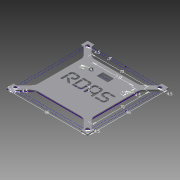
# Autodesk Inventor part: BattHolder
Saved by Autodesk Inventor 2014 SP1 (Build 180222100, 222)
## iProperties
Created: 2015-03-30
Part Number: BattHolder
Material: Generic
Document SubType Name: Modeling
Designer: Erin
Density: 1 g/cm^3
Appearance: Default
Author: Erin
Autodesk Inventor part; units mm, degrees
ref_plane "YZ Plane" through (0, 0, 0) normal (1, 0, 0) x (0, 1, 0)
ref_plane "XZ Plane" through (0, 0, 0) normal (0, 1, 0) x (-1, 0, 0)
ref_plane "XY Plane" through (0, 0, 0) normal (0, 0, 1) x (1, 0, 0)
sketch "Sketch1" plane through (0, 0, 0) normal (0, 0, 1) x (1, 0, 0)
  line L0 (-48, 48) -> (48, 48) construction
  line L1 (48, 48) -> (48, -48) construction
  line L2 (48, -48) -> (-48, -48) construction
  line L3 (-48, -48) -> (-48, 48) construction
  circle A0 centre (-45, 45) radius 2.25
  circle A1 centre (45, 45) radius 2.25
  line L4 (45, 45) -> (-45, 45) construction
  line L5 (-45, 45) -> (-45, -45) construction
  line L6 (-45, -45) -> (45, -45) construction
  line L7 (45, -45) -> (45, 45) construction
  circle A2 centre (45, -45) radius 2.25
  circle A3 centre (-45, -45) radius 2.25
  line L8 (-50.5, -50.5) -> (-42, -50.5)
  line L9 (-42, -50.5) -> (-42, -42)
  line L10 (-42, -42) -> (-50.5, -42)
  line L11 (-50.5, -42) -> (-50.5, -50.5)
  line L12 (0, 0) -> (-48, -48) construction
  line L13 (-35, 35) -> (35, 35)
  line L14 (35, 35) -> (35, -35)
  line L15 (35, -35) -> (-35, -35)
  line L16 (-35, -35) -> (-35, 35)
  line L17 (-2.4749, 2.4749) -> (2.4749, -2.4749)
  line L18 (2.4749, -2.4749) -> (-42.5251, -47.4749)
  line L19 (-42.5251, -47.4749) -> (-47.4749, -42.5251)
  line L20 (-47.4749, -42.5251) -> (-2.4749, 2.4749)
  line L21 (0, 0) -> (-45, -45) construction
  line L22 (-25, 30) -> (25, 30)
  line L23 (25, 30) -> (25, 15)
  line L24 (25, 15) -> (-25, 15)
  line L25 (-25, 15) -> (-25, 30)
  line L26 (-25, 22.5) -> (25, 22.5) construction
  circle A4 centre (-28, 22.1227) radius 2.25
  circle A5 centre (28, 22.1227) radius 2.25
  point P0 (0, 48)
  point P1 (48, 0)
  point P2 (35, 0)
  point P3 (0, 35)
  point P4 (0, 30)
  dimension "d0" = 96
  dimension "d1" = 96
  dimension "d2" = 4.5
  dimension "d3" = 4.5
  dimension "d4" = 3
  dimension "d5" = 4.5
  dimension "d6" = 4.5
  dimension "d9" = 3
  dimension "d10" = 3
  dimension "d11" = 70
  dimension "d12" = 70
  dimension "d13" = 7
  dimension "d14" = 0
  dimension "d23" = 5.5
  dimension "d24" = 5.5
  dimension "d27" = 15
  dimension "d28" = 50
  dimension "d29" = 4.5
  dimension "d30" = 4.5
  dimension "d31" = 3
  dimension "d32" = 3
  dimension "d33" = 5
  constraints: 54 end point, 12 parallel, 9 midpoint, 6 centre point, 6 perpendicular, 4 coincident, 4 horizontal, 3 vertical alignment, 2 horizontal alignment, 1 collinear, 3 other
  measures "d0" distance of L1.end L2.end
  measures "d1" distance of L0.end L1.end
  measures "d2" diameter of A0
  measures "d3" diameter of A1
  measures "d4" distance between parallel lines of L4 L0
  measures "d5" diameter of A2
  measures "d6" diameter of A3
  measures "d9" distance from line of A3.centre L10
  measures "d10" distance from line of A3.centre L9
  measures "d11" distance of L13.start L13.end
  measures "d12" distance of L13.end L14.end
  measures "d13" distance of L17.start L17.end
  measures "d14" distance from line of L5.end L19
  measures "d23" distance from line of L11 A3.centre
  measures "d24" distance from line of A3.centre L8
  measures "d27" distance of L22.end L23.end
  measures "d28" distance of L22.start L22.end
  measures "d29" diameter of A4
  measures "d30" diameter of A5
  measures "d31" distance from line of A4.centre L25
  measures "d32" distance from line of A5.centre L23
  measures "d33" distance between parallel lines of L22 L13
extrude "Extrusion1" add sketch "Sketch1" along normal blind 1.5 contours L20 L17 L18 L15 L16 | L16 L13 L14 L15 L18 L17 L20 | L22 L23 L24 L25 | A4 | A5
extrude "Extrusion2" add sketch "Sketch1" along normal blind 1.5 contours A3 L19 | A3 L19 L20 L10 L9 L18 | A3 L19 L18 L9 L8 L11 L10 L20 | L20 L16 L15 L18 L9 L10 | L20 L17 L18 L15 L16 picked at (-45.2318, -44.2867)
extrude "Extrusion3" cut sketch "Sketch1" along normal blind 10 contours A3 L19 | L19 A3
mirror "Mirror1" about plane through (0, 0, 0) normal (1, 0, 0) of "Extrusion2", "Extrusion3"
mirror "Mirror2" about plane through (0, 0, 0) normal (0, 1, 0) of "Extrusion2", "Extrusion3", "Mirror1"
fillet "Fillet2" radius 10 8 edges at (-35, -30.0503, 0.75) (-35, 30.0503, 0.75) (35, 30.0503, 0.75) (35, -30.0503, 0.75) (-30.0503, -35, 0.75) (30.0503, -35, 0.75) (30.0503, 35, 0.75) (-30.0503, 35, 0.75)
sketch "Sketch2" plane through (0, 0, 1.5) normal (0, 0, 1) x (1, 0, 0)
  line L0 (-28.3958, 7.9828) -> (28.458, 7.9828) construction
  line L1 (28.458, 7.9828) -> (28.458, -7.0172) construction
  line L2 (28.458, -7.0172) -> (-28.3958, -7.0172) construction
  line L3 (-28.3958, -7.0172) -> (-28.3958, 7.9828) construction
  line L4 (25.9081, 35) -> (-25.9081, 35) projected
  line L5 (-6.9, 26) -> (6.9, 26)
  line L6 (6.9, 26) -> (6.9, 18.2)
  line L7 (6.9, 18.2) -> (-6.9, 18.2)
  line L8 (-6.9, 18.2) -> (-6.9, 26)
  circle A0 centre (-16.9, 22.1) radius 2.9
  line L9 (-6.9, 22.1) -> (6.9, 22.1) construction
  spline S0 degree 2 poles (-17.7357, 2.8471) (-17.7357, 2.3566) (-18.4112, 1.6626) (-18.9202, 1.6626) knots 0 0 0 1 2 2 2
  line L10 (-18.9202, 1.6626) -> (-20.8912, 1.6626)
  line L11 (-20.8912, 1.6626) -> (-20.8912, -0.7063)
  line L12 (-20.8912, -0.7063) -> (-18.9202, -0.7063)
  spline S1 degree 2 poles (-18.9202, -0.7063) (-18.1892, -0.7063) (-16.8844, -0.1511) (-15.922, 0.8113) (-15.3668, 2.116) (-15.3668, 2.8471) knots 0 0 0 1 2 3 4 4 4
  line L13 (-15.3668, 2.8471) -> (-15.3668, 4.4294)
  spline S2 degree 2 poles (-15.3668, 4.4294) (-15.3668, 5.1605) (-15.922, 6.4652) (-16.8844, 7.4276) (-18.1892, 7.9828) (-18.9202, 7.9828) knots 0 0 0 1 2 3 4 4 4
  line L14 (-18.9202, 7.9828) -> (-20.8912, 7.9828)
  line L15 (-20.8912, 7.9828) -> (-20.8912, 5.6139)
  line L16 (-20.8912, 5.6139) -> (-18.9202, 5.6139)
  spline S3 degree 2 poles (-18.9202, 5.6139) (-18.4112, 5.6139) (-17.7357, 4.9199) (-17.7357, 4.4294) knots 0 0 0 1 2 2 2
  line L17 (-17.7357, 4.4294) -> (-17.7357, 2.8471)
  line L18 (-24.8425, -7.0172) -> (-27.2114, -7.0172)
  line L19 (-27.2114, -7.0172) -> (-27.2114, 1.6626)
  line L20 (-27.2114, 1.6626) -> (-24.8425, 1.6626)
  line L21 (-24.8425, 1.6626) -> (-24.8425, -7.0172)
  line L22 (-15.3668, -7.0172) -> (-15.3668, -6.5268)
  line L23 (-15.3668, -6.5268) -> (-21.03, -1.4928)
  line L24 (-21.03, -1.4928) -> (-24.0559, -1.4928)
  line L25 (-24.0559, -1.4928) -> (-24.0559, -1.9833)
  line L26 (-24.0559, -1.9833) -> (-18.365, -7.0172)
  line L27 (-18.365, -7.0172) -> (-15.3668, -7.0172)
  spline S4 degree 2 poles (-23.658, 5.6139) (-24.1484, 5.6139) (-24.8425, 4.9199) (-24.8425, 4.4294) knots 0 0 0 1 2 2 2
  line L28 (-24.8425, 4.4294) -> (-24.8425, 2.4584)
  line L29 (-24.8425, 2.4584) -> (-27.2114, 2.4584)
  line L30 (-27.2114, 2.4584) -> (-27.2114, 4.4294)
  spline S5 degree 2 poles (-27.2114, 4.4294) (-27.2114, 5.1605) (-26.6562, 6.4652) (-25.6938, 7.4276) (-24.389, 7.9828) (-23.658, 7.9828) knots 0 0 0 1 2 3 4 4 4
  line L31 (-23.658, 7.9828) -> (-21.687, 7.9828)
  line L32 (-21.687, 7.9828) -> (-21.687, 5.6139)
  line L33 (-21.687, 5.6139) -> (-23.658, 5.6139)
  spline S6 degree 2 poles (-4.7067, -4.6483) (-4.1978, -4.6483) (-3.5223, -3.9543) (-3.5223, -3.4639) knots 0 0 0 1 2 2 2
  line L34 (-3.5223, -3.4639) -> (-3.5223, 1.6719)
  line L35 (-3.5223, 1.6719) -> (-1.1534, 1.6719)
  line L36 (-1.1534, 1.6719) -> (-1.1534, -3.4639)
  spline S7 degree 2 poles (-1.1534, -3.4639) (-1.1534, -4.1949) (-1.7086, -5.4996) (-2.671, -6.462) (-3.9757, -7.0172) (-4.7067, -7.0172) knots 0 0 0 1 2 3 4 4 4
  line L37 (-4.7067, -7.0172) -> (-6.6777, -7.0172)
  line L38 (-6.6777, -7.0172) -> (-6.6777, -4.6483)
  line L39 (-6.6777, -4.6483) -> (-4.7067, -4.6483)
  line L40 (-12.9979, 4.8273) -> (-10.629, 4.8273)
  line L41 (-10.629, 4.8273) -> (-10.629, -3.8618)
  line L42 (-10.629, -3.8618) -> (-12.9979, -3.8618)
  line L43 (-12.9979, -3.8618) -> (-12.9979, 4.8273)
  spline S8 degree 2 poles (-3.5223, 4.4294) (-3.5223, 4.9199) (-4.1978, 5.6139) (-4.7067, 5.6139) knots 0 0 0 1 2 2 2
  line L44 (-4.7067, 5.6139) -> (-6.6777, 5.6139)
  line L45 (-6.6777, 5.6139) -> (-6.6777, 7.9828)
  line L46 (-6.6777, 7.9828) -> (-4.7067, 7.9828)
  spline S9 degree 2 poles (-4.7067, 7.9828) (-3.9757, 7.9828) (-2.671, 7.4276) (-1.7086, 6.4652) (-1.1534, 5.1605) (-1.1534, 4.4294) knots 0 0 0 1 2 3 4 4 4
  line L47 (-1.1534, 4.4294) -> (-1.1534, 2.4584)
  line L48 (-1.1534, 2.4584) -> (-3.5223, 2.4584)
  line L49 (-3.5223, 2.4584) -> (-3.5223, 4.4294)
  line L50 (-7.4735, 7.9828) -> (-7.4735, 5.6139)
  line L51 (-7.4735, 5.6139) -> (-12.9979, 5.6139)
  line L52 (-12.9979, 5.6139) -> (-12.9979, 7.9828)
  line L53 (-12.9979, 7.9828) -> (-7.4735, 7.9828)
  line L54 (-7.4735, -4.6483) -> (-7.4735, -7.0172)
  line L55 (-7.4735, -7.0172) -> (-12.9979, -7.0172)
  line L56 (-12.9979, -7.0172) -> (-12.9979, -4.6483)
  line L57 (-12.9979, -4.6483) -> (-7.4735, -4.6483)
  line L58 (6.7399, -1.4928) -> (6.7399, -3.8618)
  line L59 (6.7399, -3.8618) -> (4.7689, -3.8618)
  spline S10 degree 2 poles (4.7689, -3.8618) (4.2785, -3.8618) (3.5844, -4.5558) (3.5844, -5.0462) knots 0 0 0 1 2 2 2
  line L60 (3.5844, -5.0462) -> (3.5844, -7.0172)
  line L61 (3.5844, -7.0172) -> (1.2155, -7.0172)
  line L62 (1.2155, -7.0172) -> (1.2155, 1.6626)
  line L63 (1.2155, 1.6626) -> (3.5844, 1.6626)
  line L64 (3.5844, 1.6626) -> (3.5844, -0.3084)
  spline S11 degree 2 poles (3.5844, -0.3084) (3.5844, -0.7988) (4.2785, -1.4928) (4.7689, -1.4928) knots 0 0 0 1 2 2 2
  line L65 (4.7689, -1.4928) -> (6.7399, -1.4928)
  line L66 (7.5357, -3.8618) -> (7.5357, -1.4928)
  line L67 (7.5357, -1.4928) -> (9.5067, -1.4928)
  spline S12 degree 2 poles (9.5067, -1.4928) (10.0157, -1.4928) (10.6912, -0.7988) (10.6912, -0.3084) knots 0 0 0 1 2 2 2
  line L68 (10.6912, -0.3084) -> (10.6912, 1.6626)
  line L69 (10.6912, 1.6626) -> (13.0601, 1.6626)
  line L70 (13.0601, 1.6626) -> (13.0601, -7.0172)
  line L71 (13.0601, -7.0172) -> (10.6912, -7.0172)
  line L72 (10.6912, -7.0172) -> (10.6912, -5.0462)
  spline S13 degree 2 poles (10.6912, -5.0462) (10.6912, -4.5558) (10.0157, -3.8618) (9.5067, -3.8618) knots 0 0 0 1 2 2 2
  line L73 (9.5067, -3.8618) -> (7.5357, -3.8618)
  line L74 (3.5844, 2.4584) -> (1.2155, 2.4584)
  line L75 (1.2155, 2.4584) -> (1.2155, 4.4294)
  spline S14 degree 2 poles (1.2155, 4.4294) (1.2155, 5.1605) (1.7707, 6.4652) (2.7331, 7.4276) (4.0379, 7.9828) (4.7689, 7.9828) knots 0 0 0 1 2 3 4 4 4
  line L76 (4.7689, 7.9828) -> (6.7399, 7.9828)
  line L77 (6.7399, 7.9828) -> (6.7399, 5.6139)
  line L78 (6.7399, 5.6139) -> (4.7689, 5.6139)
  spline S15 degree 2 poles (4.7689, 5.6139) (4.2785, 5.6139) (3.5844, 4.9199) (3.5844, 4.4294) knots 0 0 0 1 2 2 2
  line L79 (3.5844, 4.4294) -> (3.5844, 2.4584)
  line L80 (7.5357, 5.6139) -> (7.5357, 7.9828)
  line L81 (7.5357, 7.9828) -> (9.5067, 7.9828)
  spline S16 degree 2 poles (9.5067, 7.9828) (10.2377, 7.9828) (11.5425, 7.4276) (12.5049, 6.4652) (13.0601, 5.1605) (13.0601, 4.4294) knots 0 0 0 1 2 3 4 4 4
  line L82 (13.0601, 4.4294) -> (13.0601, 2.4584)
  line L83 (13.0601, 2.4584) -> (10.6912, 2.4584)
  line L84 (10.6912, 2.4584) -> (10.6912, 4.4294)
  spline S17 degree 2 poles (10.6912, 4.4294) (10.6912, 4.9199) (10.0157, 5.6139) (9.5067, 5.6139) knots 0 0 0 1 2 2 2
  line L85 (9.5067, 5.6139) -> (7.5357, 5.6139)
  spline S18 degree 2 poles (24.9046, -3.4639) (24.9046, -3.9543) (24.2291, -4.6483) (23.7202, -4.6483) knots 0 0 0 1 2 2 2
  line L86 (23.7202, -4.6483) -> (21.7492, -4.6483)
  line L87 (21.7492, -4.6483) -> (21.7492, -7.0172)
  line L88 (21.7492, -7.0172) -> (23.7202, -7.0172)
  spline S19 degree 2 poles (23.7202, -7.0172) (24.4512, -7.0172) (25.7559, -6.462) (26.7183, -5.4996) (27.2735, -4.1949) (27.2735, -3.4639) knots 0 0 0 1 2 3 4 4 4
  line L89 (27.2735, -3.4639) -> (27.2735, -1.8815)
  spline S20 degree 2 poles (27.2735, -1.8815) (27.2735, -1.1505) (26.7183, 0.1543) (25.7559, 1.1167) (24.4512, 1.6719) (23.7202, 1.6719) knots 0 0 0 1 2 3 4 4 4
  line L90 (23.7202, 1.6719) -> (21.7492, 1.6719)
  line L91 (21.7492, 1.6719) -> (21.7492, -0.697)
  line L92 (21.7492, -0.697) -> (23.7202, -0.697)
  spline S21 degree 2 poles (23.7202, -0.697) (24.2291, -0.697) (24.9046, -1.3911) (24.9046, -1.8815) knots 0 0 0 1 2 2 2
  line L93 (24.9046, -1.8815) -> (24.9046, -3.4639)
  spline S22 degree 2 poles (17.7979, 4.4294) (17.7979, 4.9199) (18.4919, 5.6139) (18.9823, 5.6139) knots 0 0 0 1 2 2 2
  line L94 (18.9823, 5.6139) -> (20.9533, 5.6139)
  line L95 (20.9533, 5.6139) -> (20.9533, 7.9828)
  line L96 (20.9533, 7.9828) -> (18.9823, 7.9828)
  spline S23 degree 2 poles (18.9823, 7.9828) (18.2513, 7.9828) (16.9466, 7.4276) (15.9842, 6.4652) (15.429, 5.1605) (15.429, 4.4294) knots 0 0 0 1 2 3 4 4 4
  line L97 (15.429, 4.4294) -> (15.429, 2.8563)
  spline S24 degree 2 poles (15.429, 2.8563) (15.429, 2.1253) (15.9842, 0.8205) (16.9466, -0.1418) (18.2513, -0.697) (18.9823, -0.697) knots 0 0 0 1 2 3 4 4 4
  line L98 (18.9823, -0.697) -> (20.9533, -0.697)
  line L99 (20.9533, -0.697) -> (20.9533, 1.6719)
  line L100 (20.9533, 1.6719) -> (18.9823, 1.6719)
  spline S25 degree 2 poles (18.9823, 1.6719) (18.4919, 1.6719) (17.7979, 2.3659) (17.7979, 2.8563) knots 0 0 0 1 2 2 2
  line L101 (17.7979, 2.8563) -> (17.7979, 4.4294)
  line L102 (21.7492, 5.6139) -> (21.7492, 7.9828)
  line L103 (21.7492, 7.9828) -> (27.2735, 7.9828)
  line L104 (27.2735, 7.9828) -> (27.2735, 5.6139)
  line L105 (27.2735, 5.6139) -> (21.7492, 5.6139)
  line L106 (15.429, -7.0172) -> (15.429, -4.6483)
  line L107 (15.429, -4.6483) -> (20.9533, -4.6483)
  line L108 (20.9533, -4.6483) -> (20.9533, -7.0172)
  line L109 (20.9533, -7.0172) -> (15.429, -7.0172)
  point P0 (0, 0)
  point P1 (0, 26)
  dimension "d36" = 5.8
  dimension "d37" = 13.8
  dimension "d38" = 7.8
  dimension "d39" = 10
  dimension "d40" = 9
  constraints: 10 end point, 3 midpoint, 2 parallel, 1 centre point, 1 horizontal, 1 perpendicular, 1 point on line, 1 vertical alignment, 2 other
  measures "d36" diameter of A0
  measures "d37" distance of L6.end L7.end
  measures "d38" distance of L5.end L6.end
  measures "d39" distance from line of A0.centre L8
  measures "d40" distance between parallel lines of L5 L4
extrude "Extrusion4" cut sketch "Sketch2" against normal blind 10 contours L17 S3 L16 L15 L14 S2 L13 S1 L12 L11 L10 S0 | L18 L19 L20 L21 | L27 L26 L25 L24 L23 L22 | S4 L28 L29 L30 S5 L31 L32 L33 | S6 L34 L35 L36 S7 L37 L38 L39 | L40 L41 L42 L43 | S8 L44 L45 L46 S9 L47 L48 L49 | L50 L51 L52 L53 | L54 L55 L56 L57 | L58 L59 S10 L60 L61 L62 L63 L64 S11 L65 | L66 L67 S12 L68 L69 L70 L71 L72 S13 L73 | L74 L75 S14 L76 L77 L78 S15 L79 | L80 L81 S16 L82 L83 L84 S17 L85 | L93 S21 L92 L91 L90 S20 L89 S19 L88 L87 L86 S18 | L101 S25 L100 L99 L98 S24 L97 S23 L96 L95 L94 S22 | L102 L103 L104 L105 | L106 L107 L108 L109
extrude "Extrusion5" [suppressed]
extrude "Extrusion6" cut sketch "Sketch2" against normal blind 10 contours L5 L6 L7 L8 | A0
body "Solid1"
